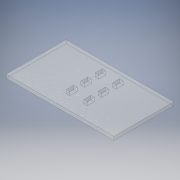
# Autodesk Inventor part: phone_holder_back
Saved by Autodesk Inventor 2019 (Build 230136000, 136)
## iProperties
Created: 2019-02-17
Part Number: phone_holder_back
Material: Acrylic, Clear
Document SubType Name: Modeling
Designer: suchanek
Density: 1.19 g/cm^3
Appearance: Transparent - Clear
Author: suchanek
Autodesk Inventor part; units mm, degrees
ref_plane "YZ Plane" through (0, 0, 0) normal (1, 0, 0) x (0, 1, 0)
ref_plane "XZ Plane" through (0, 0, 0) normal (0, 1, 0) x (-1, 0, 0)
ref_plane "XY Plane" through (0, 0, 0) normal (0, 0, 1) x (1, 0, 0)
sketch "Sketch2" plane through (0, 0, 0) normal (0, 1, 0) x (-1, 0, 0)
  line L0 (90, 50) -> (-90, 50)
  line L1 (-90, 50) -> (-90, -50)
  line L2 (-90, -50) -> (90, -50)
  line L3 (90, -50) -> (90, 50)
  line L4 (90, 50) -> (-90, -50) construction
  line L5 (-90, 50) -> (90, -50) construction
  line L6 (11.5, -38) -> (17.5, -38)
  line L7 (17.5, -38) -> (17.5, -26)
  line L8 (17.5, -26) -> (11.5, -26)
  line L9 (11.5, -26) -> (11.5, -38)
  line L10 (11.5, -14) -> (17.5, -14)
  line L11 (17.5, -14) -> (17.5, -2)
  line L12 (17.5, -2) -> (11.5, -2)
  line L13 (11.5, -2) -> (11.5, -14)
  line L14 (11.5, 10) -> (17.5, 10)
  line L15 (17.5, 10) -> (17.5, 22)
  line L16 (17.5, 22) -> (11.5, 22)
  line L17 (11.5, 22) -> (11.5, 10)
  line L18 (-17.5, -38) -> (-11.5, -38)
  line L19 (-11.5, -38) -> (-11.5, -26)
  line L20 (-11.5, -26) -> (-17.5, -26)
  line L21 (-17.5, -26) -> (-17.5, -38)
  line L22 (-17.5, -14) -> (-11.5, -14)
  line L23 (-11.5, -14) -> (-11.5, -2)
  line L24 (-11.5, -2) -> (-17.5, -2)
  line L25 (-17.5, -2) -> (-17.5, -14)
  line L26 (-17.5, 10) -> (-11.5, 10)
  line L27 (-11.5, 10) -> (-11.5, 22)
  line L28 (-11.5, 22) -> (-17.5, 22)
  line L29 (-17.5, 22) -> (-17.5, 10)
  line L30 (0, 0) -> (0, -11.4718)
  dimension "d52" = 180
  dimension "d53" = 100
  dimension "d54" = 12
  dimension "d55" = 6
  dimension "d58" = 24
  dimension "d61" = 29
  dimension "d65" = 12
  constraints: 62 end point, 4 parallel, 3 horizontal, 2 midpoint, 2 perpendicular, 2 vertical, 41 other
  measures "d52" distance of L2.end L1.end
  measures "d53" distance of L1.end L0.end
  measures "d54" distance of L8.end L6.start
  measures "d55" distance of L6.start L6.end
  measures "d58" distance of L6.start L10.start
  measures "d61" distance of L6.start L18.start
  measures "d65" distance between parallel lines of L2 L6
extrude "Extrusion2" add sketch "Sketch2" along normal blind 6
body "Solid2"
